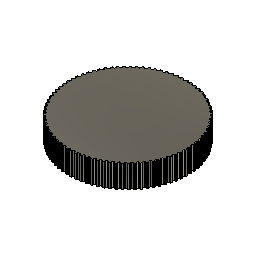
gear_83z (Autodesk Fusion 360 design; units mm, degrees)
Autodesk Fusion 360 part; units mm, degrees
sketch "Sketch1" plane through (0, 0, 0) normal (0, 0, 1) x (1, 0, 0) in component "gt2 pulley"
  circle A0 centre (0, 0) radius 26.4197 construction
  circle A1 centre (0, 0) radius 25.4157 construction
  line L0 (0, 0) -> (0, 26.4197) construction
  line L1 (0, 0) -> (0.9998, 26.4008) construction
  line L2 (0, 0) -> (1.4047, 26.3823) construction
  circle A2 centre (0, 0) radius 26.1657 construction
  arc A3 (0.3962, 26.0294) -> (0.4733, 25.7319) centre (1.3912, 26.1287) ccw
  circle A4 centre (0, 0) radius 26.0157 construction
  arc A5 (0.2483, 26.1645) -> (0, 26.1657) centre (0, 0) ccw
  arc A6 (0.3962, 26.0294) -> (0.2483, 26.1645) centre (0.2469, 26.0145) ccw
  arc A7 (0.4733, 25.7319) -> (0.9618, 25.3975) centre (0.9828, 25.9521) ccw
  arc A8 (0, 26.1657) -> (-0.2483, 26.1645) centre (0, 0) ccw
  arc A9 (-0.2483, 26.1645) -> (-0.3962, 26.0294) centre (-0.2469, 26.0145) ccw
  arc A10 (-0.4733, 25.7319) -> (-0.3962, 26.0294) centre (-1.3912, 26.1287) ccw
  arc A11 (-0.9622, 25.3975) -> (-0.4733, 25.7319) centre (-0.9828, 25.9521) ccw
  arc A12 (0.9618, 25.3975) -> (-0.9618, 25.3975) centre (0, 0) ccw
  point P0 (1.3912, 26.1287)
  point P1 (0, 26.1657)
  dimension "d18" = 52.8394
  dimension "d19" = 2.169
  dimension "d22" = 1.004
  dimension "d24" = 0.75
  dimension "d26" = 1
  dimension "d27" = 0.15
  dimension "d28" = 0.15
  dimension "d47" = 0.555
  dimension "d52" = 3.812
  constraint coincident A0.centre A1.centre
  constraint coincident A0 L0.end
  constraint vertical L0
  constraint coincident A0 L1.end
  constraint coincident A0 L2.end
  constraint concentric A1 A2
  constraint coincident A1 A7.end
  constraint coincident L1 A7.end
  constraint coincident A2 P0
  constraint coincident L2 P0
  constraint coincident P0 A3.centre
  constraint coincident A2 P1
  constraint coincident L0 P1
  constraint concentric A2 A4
  constraint coincident P1 A5.end
  constraint coincident A4 A6.centre
  constraint coincident A3.start A6.start
  constraint tangent A3 A6
  constraint tangent A3 A7
  constraint symmetric L0 A7.end A12.end
  constraint symmetric L0 A3.start A9.end
  constraint symmetric L0 A3.end A10.start
  constraint symmetric L0 A3 A10
  constraint symmetric L0 A5.start A8.end
  constraint symmetric L0 P1 A5.end
  constraint symmetric L0 A5 A8
  constraint symmetric L0 A6 A9
  constraint symmetric L0 A7 A11
  constraint coincident A1 A11.start
  constraint tangent A1 A7
  constraint coincident L1 A7.centre
  measures "d18" diameter of A0
  measures "d19" angle of L0 L1
  measures "d22" distance of A0 A1
  measures "d24" distance of A1 A2
  measures "d26" radius of A3
  measures "d27" distance of A2 A4
  measures "d28" radius of A6
  measures "d47" radius of A7
extrude "Extrude1" add sketch "Sketch1" along normal blind 10 makes body 1
pattern_circular "C-Pattern1" count 83 over 360 about axis through (0, 0, 1.75) along (0, 0, 1) of bodies 1 makes body 2 at (-1.1754, 25.3885, 3.3333) makes body 3 at (-4.5716, 25.0012, 6.6667) makes body 4 at (-6.4493, 24.5838, 6.6667) makes body 5 at (-8.2901, 24.0257, 6.6667) makes body 6 at (-8.6927, 23.8829, 6.6667) makes body 7 at (-10.4741, 23.1571, 3.3333) makes body 8 at (-12.1954, 22.2987, 3.3333) makes body 9 at (-13.8469, 21.3125, 3.3333) makes body 10 at (-15.4191, 20.2042, 6.6667) makes body 11 at (-17.532, 18.4008, 6.6667) makes body 12 at (-19.297, 16.5404, 6.6667) makes body 13 at (-20.4926, 15.0336, 6.6667) makes body 14 at (-20.7424, 14.6871, 3.3333) makes body 15 at (-22.5257, 11.7709, 6.6667) makes body 16 at (-23.3514, 10.0336, 6.6667) makes body 17 at (-23.5167, 9.6397, 3.3333) makes body 18 at (-24.4283, 7.0156, 6.6667) makes body 19 at (-24.7016, 5.9825, 3.3333) makes body 20 at (-25.281, 2.6138, 6.6667) makes body 21 at (-25.3806, 1.3353, 6.6667) makes body 22 at (-25.386, -1.2291, 6.6667) makes body 23 at (-25.3617, -1.6556, 3.3333) makes body 24 at (-25.0296, -4.4136, 6.6667) makes body 25 at (-24.4574, -6.9134, 6.6667) makes body 26 at (-24.3377, -7.3235, 3.3333) makes body 27 at (-23.3931, -9.9358, 6.6667) makes body 28 at (-22.2728, -12.2426, 6.6667) makes body 29 at (-21.3993, -13.7124, 6.6667) makes body 30 at (-21.0466, -14.2478, 6.6667) makes body 31 at (-19.0863, -16.7831, 6.6667) makes body 32 at (-18.657, -17.2591, 3.3333) makes body 33 at (-16.1723, -19.6065, 6.6667) makes body 34 at (-15.1627, -20.3973, 6.6667) makes body 35 at (-14.2919, -21.0167, 3.3333) makes body 36 at (-11.3425, -22.7444, 6.6667) makes body 37 at (-10.9586, -22.9318, 6.6667) makes body 38 at (-7.7823, -24.1949, 6.6667) makes body 39 at (-5.9302, -24.7142, 6.6667) makes body 40 at (-4.6761, -24.9819, 6.6667) makes body 41 at (-2.1349, -25.3259, 6.6667) makes body 42 at (-0.2134, -25.4148, 6.6667) makes body 43 at (1.7093, -25.3582, 6.6667) makes body 44 at (2.1353, -25.3259, 3.3333) makes body 45 at (5.5144, -24.8103, 6.6667) makes body 46 at (6.5524, -24.5566, 6.6667) makes body 47 at (7.7827, -24.1948, 3.3333) makes body 48 at (10.1812, -23.2874, 6.6667) makes body 49 at (12.6619, -22.0371, 6.6667) makes body 50 at (14.2923, -21.0164, 6.6667) makes body 51 at (15.8408, -19.8753, 6.6667) makes body 52 at (16.8231, -19.051, 6.6667) makes body 53 at (18.6572, -17.2588, 6.6667) makes body 54 at (19.9091, -15.7984, 6.6667) makes body 55 at (20.6806, -14.774, 6.6667) makes body 56 at (21.7387, -13.1677, 6.6667) makes body 57 at (22.6723, -11.4859, 6.6667) makes body 58 at (23.1351, -10.5227, 3.3333) makes body 59 at (24.1453, -7.9349, 6.6667) makes body 60 at (24.822, -5.4615, 6.6667) makes body 61 at (24.9103, -5.0435, 3.3333) makes body 62 at (25.2204, -3.1451, 6.6667) makes body 63 at (25.4143, 0.2676, 6.6667) makes body 64 at (25.3213, 2.1889, 6.6667) makes body 65 at (25.2069, 3.2514, 6.6667) makes body 66 at (24.751, 5.7749, 6.6667) makes body 67 at (24.5974, 6.3973, 3.3333) makes body 68 at (24.0432, 8.2392, 3.3333) makes body 69 at (22.7201, 11.391, 6.6667) makes body 70 at (22.2212, 12.336, 6.6667) makes body 71 at (20.7422, 14.6874, 6.6667) makes body 72 at (19.572, 16.2141, 6.6667) makes body 73 at (18.2897, 17.6478, 6.6667) makes body 74 at (17.9905, 17.9528, 3.3333) makes body 75 at (15.4188, 20.2045, 6.6667) makes body 76 at (15.077, 20.4608, 3.3333) makes body 77 at (12.1951, 22.2989, 6.6667) makes body 78 at (11.8185, 22.5007, 3.3333) makes body 79 at (8.6923, 23.8831, 6.6667) makes body 80 at (7.0668, 24.4135, 6.6667) makes body 81 at (4.9908, 24.9209, 6.6667) makes body 82 at (4.5712, 25.0013, 3.3333) makes body 83 at (1.3885, 25.3778, 6.6667)
sketch "Sketch2" plane through (0, 0, 10) normal (0, 0, 1) x (-1, 0, 0)
  arc A0 (-9.9868, -24.0406) -> (-9.8993, -24.2208) centre (-9.8426, -24.0819) ccw
  arc A1 (-9.8993, -24.2208) -> (-9.4379, -24.4043) centre (0, 0) ccw
  arc A2 (-9.4379, -24.4043) -> (-9.2506, -24.3334) centre (-9.3838, -24.2644) ccw
  arc A3 (-9.0689, -24.0854) -> (-9.2506, -24.3334) centre (-8.3626, -24.7934) ccw
  arc A4 (-8.4915, -23.9552) -> (-9.0689, -24.0854) centre (-8.6769, -24.4783) ccw
  arc A5 (-10.2789, -23.2444) -> (-8.4915, -23.9552) centre (0, 0) ccw
  arc A6 (-9.9486, -23.7356) -> (-10.2789, -23.2444) centre (-10.5033, -23.752) ccw
  arc A7 (-9.9868, -24.0406) -> (-9.9486, -23.7356) centre (-10.9481, -23.7652) ccw
  circle A8 centre (0, 0) radius 25.4157
  constraint concentric A1 A8
extrude "Extrude2" add sketch "Sketch2" against normal blind 10 contours A5 A8 bodies 1 2 3 4 5 6 7 8 9 10 11 12 13 14 15 16 17 18 19 20 21 22 23 24 25 26 27 28 29 30 31 32 33 34 35 36 37 38 39 40 41 42 43 44 45 46 47 48 49 50 51 52 53 54 55 56 57 58 59 60 61 62 63 64 65 66 67 68 69 70 71 72 73 74 75 76 77 78 79 80 81 82 83
extrude "Extrude4" [suppressed] in component "gt2 pulley"
pattern_circular "C-Pattern7" [suppressed] in component "gt2 pulley"
extrude "Extrude3" [suppressed] in component "gt2 pulley"
pattern_circular "C-Pattern6" [suppressed] in component "gt2 pulley"
extrude "Extrude2'" [suppressed] in component "gt2 pulley"
pattern_circular "C-Pattern5" [suppressed] in component "gt2 pulley"
extrude "Extrude1'" [suppressed] in component "gt2 pulley"
pattern_circular "C-Pattern4" [suppressed] in component "gt2 pulley"
pattern_circular "C-Pattern3" [suppressed] in component "gt2 pulley"
pattern_circular "C-Pattern2" [suppressed] in component "gt2 pulley"
pattern_circular "C-Pattern1'" [suppressed] in component "gt2 pulley"
copy_body "Body->Comp1" [suppressed] in component "Component"
copy_body "Body->Comp2" [suppressed] in component "Component'"
copy_body "Body->Comp3" [suppressed] in component "Component''"
copy_body "Body->Comp4" [suppressed] in component "Component'''"
copy_body "Body->Comp5" [suppressed] in component "Component''''"
copy_body "Body->Comp6" [suppressed] in component "Component'''''"
copy_body "Body->Comp7" [suppressed] in component "Component''''''"
copy_body "Body->Comp8" [suppressed] in component "Component'''''''"
copy_body "Body->Comp9" [suppressed] in component "Component''''''''"
copy_body "Body->Comp10" [suppressed] in component "Component'''''''''"
copy_body "Body->Comp11" [suppressed] in component "Component''''''''''"
copy_body "Body->Comp12" [suppressed] in component "Component'''''''''''"
copy_body "Body->Comp13" [suppressed] in component "Component''''''''''''"
copy_body "Body->Comp14" [suppressed] in component "Component'''''''''''''"
copy_body "Body->Comp15" [suppressed] in component "Component''''''''''''''"
copy_body "Body->Comp16" [suppressed] in component "Component'''''''''''''''"
copy_body "Body->Comp17" [suppressed] in component "Component''''''''''''''''"
copy_body "Body->Comp18" [suppressed] in component "Component'''''''''''''''''"
copy_body "Body->Comp19" [suppressed] in component "Component''''''''''''''''''"
copy_body "Body->Comp20" [suppressed] in component "Component'''''''''''''''''''"
component "gt2 pulley" placed x (1, 0, 0) y (0, 1, 0) z (0, 0, 1) at (0, 0, 0)
equation "NumTeeth = 83" comment "min 20"
equation "ToothPitch = 2 mm"
equation "PullyDia = NumTeeth * ToothPitch / PI"
equation "ToothAng = ( ( 360 / NumTeeth ) * 1 deg )"
equation "TransOffsetAngle = ToothAng * 0.2"
equation "Sholulder_Radius = 0.15 mm"
equation "Root_Radius = 0.555 mm"
equation "TransRadius = 1 mm"
equation "ToolHeight = 0.75 mm"
equation "PLD = 0.254 mm"
equation "d18 = PullyDia"
equation "d19 = ToothAng / 2"
equation "d22 = PLD + ToolHeight"
equation "d24 = ToolHeight"
equation "d26 = TransRadius"
equation "d27 = Sholulder_Radius"
equation "d31 = NumTeeth"
equation "d33 = NumTeeth"
equation "d35 = NumTeeth"
equation "d37 = NumTeeth"
equation "d41 = NumTeeth"
equation "d45 = NumTeeth"
equation "d47 = Root_Radius"
equation "d50 = NumTeeth"
